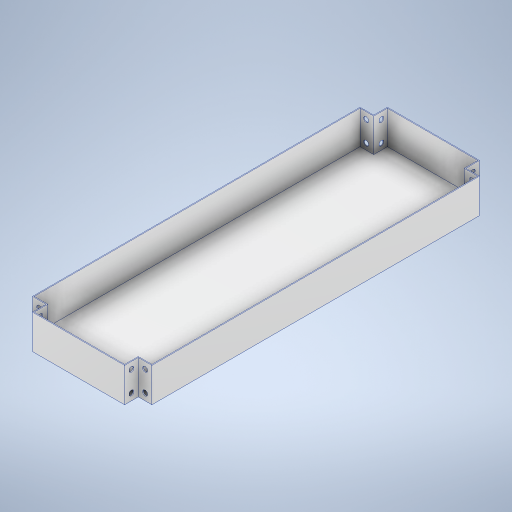
# Autodesk Inventor part: EBox-Frame
Saved by Autodesk Inventor 2023 (Build 270158000, 158)
## iProperties
Created: 2022-09-23
Part Number: EBox-Frame
Material: Aluminum 6061
Document SubType Name: Modeling
Designer: seene
Density: 2.7 g/cm^3
Appearance: Aluminum - Flat
Author: seene
Autodesk Inventor part; units mm, degrees
ref_plane "YZ Plane" through (0, 0, 0) normal (1, 0, 0) x (0, 1, 0)
ref_plane "XZ Plane" through (0, 0, 0) normal (0, 1, 0) x (-1, 0, 0)
ref_plane "XY Plane" through (0, 0, 0) normal (0, 0, 1) x (1, 0, 0)
sketch "Electronics box bottom layout" plane through (0, 0, 0) normal (0, 1, 0) x (-1, 0, 0)
  line L0 (-111.125, 304.8) -> (111.125, 304.8)
  line L1 (111.125, 304.8) -> (111.125, -304.8)
  line L2 (111.125, -304.8) -> (-111.125, -304.8)
  line L3 (-111.125, -304.8) -> (-111.125, 304.8)
  line L4 (-111.125, 304.8) -> (111.125, -304.8) construction
  line L5 (111.125, 304.8) -> (-111.125, -304.8) construction
  line L6 (-85.725, 304.8) -> (85.725, 304.8)
  line L7 (85.725, 304.8) -> (85.725, 330.2)
  line L8 (85.725, 330.2) -> (-85.725, 330.2)
  line L9 (-85.725, 330.2) -> (-85.725, 304.8)
  line L10 (-85.725, 304.8) -> (85.725, 330.2) construction
  line L11 (85.725, 304.8) -> (-85.725, 330.2) construction
  line L12 (85.725, -304.8) -> (-85.725, -304.8)
  line L13 (-85.725, -304.8) -> (-85.725, -330.2)
  line L14 (-85.725, -330.2) -> (85.725, -330.2)
  line L15 (85.725, -330.2) -> (85.725, -304.8)
  line L16 (85.725, -304.8) -> (-85.725, -330.2) construction
  line L17 (-85.725, -304.8) -> (85.725, -330.2) construction
  point P0 (0, 0)
  point P1 (0, 317.5)
  point P2 (0, -317.5)
  point P3 (-85.725, 304.8)
  dimension "d0" = 222.25
  dimension "d1" = 609.6
  dimension "d2" = 171.45
  dimension "d3" = 171.45
  dimension "d4" = 25.4
  dimension "d5" = 25.4
  constraints: 36 end point, 6 midpoint, 6 parallel, 3 horizontal, 3 perpendicular, 2 collinear, 2 vertical alignment
  measures "d0" distance of L1.end L2.end
  measures "d1" distance of L0.end L1.end
  measures "d2" distance of L14.end L13.end
  measures "d3" distance of L7.end L8.end
  measures "d4" distance of L8.end L6.start
  measures "d5" distance of L12.end L13.end
extrude "Base" add sketch "Electronics box bottom layout" along normal blind 1.5875
sketch "Sketch2" plane through (0, 1.5875, 0) normal (0, 1, 0) x (1, 0, 0)
  line L0 (-111.125, -304.8) -> (-85.725, -304.8) projected
  line L1 (-85.725, -304.8) -> (-85.725, -330.2) projected
  line L2 (-85.725, -330.2) -> (85.725, -330.2) projected
  line L3 (85.725, -330.2) -> (85.725, -304.8) projected
  line L4 (85.725, -304.8) -> (111.125, -304.8) projected
  line L5 (111.125, -304.8) -> (111.125, 304.8) projected
  line L6 (111.125, 304.8) -> (85.725, 304.8) projected
  line L7 (85.725, 304.8) -> (85.725, 330.2) projected
  line L8 (85.725, 330.2) -> (-85.725, 330.2) projected
  line L9 (-85.725, 330.2) -> (-85.725, 304.8) projected
  line L10 (-85.725, 304.8) -> (-111.125, 304.8) projected
  line L11 (-111.125, 304.8) -> (-111.125, -304.8) projected
  line L12 (-109.5375, -303.2125) -> (-84.1375, -303.2125)
  line L13 (-84.1375, -303.2125) -> (-84.1375, -328.6125)
  line L14 (-84.1375, -328.6125) -> (84.1375, -328.6125)
  line L15 (84.1375, -328.6125) -> (84.1375, -303.2125)
  line L16 (84.1375, -303.2125) -> (109.5375, -303.2125)
  line L17 (109.5375, -303.2125) -> (109.5375, 303.2125)
  line L18 (109.5375, 303.2125) -> (84.1375, 303.2125)
  line L19 (84.1375, 303.2125) -> (84.1375, 328.6125)
  line L20 (84.1375, 328.6125) -> (-84.1375, 328.6125)
  line L21 (-84.1375, 328.6125) -> (-84.1375, 303.2125)
  line L22 (-84.1375, 303.2125) -> (-109.5375, 303.2125)
  line L23 (-109.5375, 303.2125) -> (-109.5375, -303.2125)
  point P0 (0, 0)
  dimension "d8" = 1.5875
  constraints: 24 end point, 11 other
  measures "d8" distance between parallel lines of L11 L23
extrude "Walls" add sketch "Sketch2" along normal blind 61.9125
sketch "Sketch3" plane through (-85.725, 0, -330.2) normal (-1, 0, 0) x (0, 0, 1)
  line L0 (0, 63.5) -> (25.4, 63.5) projected
  line L1 (0, 0) -> (25.4, 0) projected
  line L2 (0, 0) -> (0, 63.5) projected
  point P0 (330.2, 0)
  point P1 (12.7, 50.8)
  point P2 (12.7, 12.7)
  dimension "d11" = 12.7
  dimension "d12" = 12.7
  dimension "d31" = 12.7
  dimension "d32" = 12.7
  measures "d11" distance from line of L0 point (12.7, 50.8)
  measures "d12" distance from line of L1 point (12.7, 12.7)
  measures "d31" distance from line of L2 point (12.7, 50.8)
  measures "d32" distance from line of L2 point (12.7, 12.7)
hole "Hole1" at (-85.725, 50.8, -317.5) at (-85.725, 12.7, -317.5) direction (1, 0, 0) diameter 9.525 end through all
sketch "Sketch4" plane through (-85.725, 0, -304.8) normal (0, 0, -1) x (-1, 0, 0)
  line L0 (0, 63.5) -> (25.4, 63.5) projected
  line L1 (25.4, 0) -> (25.4, 63.5) projected
  line L2 (0, 0) -> (25.4, 0) projected
  point P0 (-85.725, 0)
  point P1 (12.7, 50.8)
  point P2 (12.7, 12.7)
  dimension "d20" = 12.7
  dimension "d21" = 12.7
  dimension "d22" = 12.7
  dimension "d23" = 12.7
  measures "d20" distance from line of L0 point (12.7, 50.8)
  measures "d21" distance from line of L1 point (12.7, 50.8)
  measures "d22" distance from line of L2 point (12.7, 12.7)
  measures "d23" distance from line of L1 point (12.7, 12.7)
hole "Hole2" at (-98.425, 50.8, -304.8) at (-98.425, 12.7, -304.8) direction (0, 0, 1) diameter 9.525 end through all
pattern_linear "Rectangular Pattern1" count 2 spacing 635 along (0, 0, 1) of "Hole1" first direction both ways yes
pattern_linear "Rectangular Pattern2" count 2 spacing 196.85 along (1, 0, 0) of "Hole2"
equation "\"d2\" = d0 - 2 * d4"
equation "\"d3\" = d2"
equation "\"d5\" = d4"
equation "\"d12\" = d11"
equation "\"d32\" = d31"
body "Solid1"
